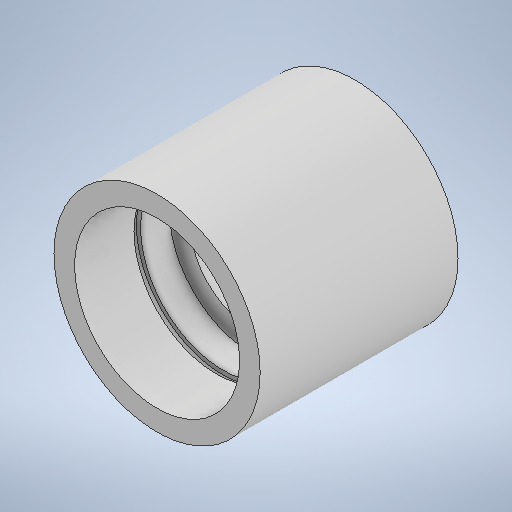
# Autodesk Inventor part: Седло для подшипника
Saved by Autodesk Inventor 2025 (Build 290162010, 162A)
## iProperties
Created: 2024-07-07
Part Number: Седло для подшипника
Material: Generic
Document SubType Name: Modeling
Designer: pokla
Density: 1 g/cm^3
Appearance: Default
Stock Number: Седло для подшипника
Author: pokla
Autodesk Inventor part; units mm, degrees
ref_plane "YZ Plane" through (0, 0, 0) normal (1, 0, 0) x (0, 1, 0)
ref_plane "XZ Plane" through (0, 0, 0) normal (0, 1, 0) x (-1, 0, 0)
ref_plane "XY Plane" through (0, 0, 0) normal (0, 0, 1) x (1, 0, 0)
sketch "Sketch6" plane through (0, 0, 0) normal (0, 0, 1) x (1, 0, 0)
  line L0 (20, 24) -> (25, 24)
  line L1 (25, 24) -> (25, -24)
  line L2 (25, -24) -> (20, -24)
  line L3 (20, -24) -> (20, -9.6)
  line L4 (15, 1) -> (20, 1)
  line L5 (20, 1) -> (20, -1) construction
  line L6 (20, -1) -> (15, -1)
  line L7 (15, -1) -> (15, 1)
  line L8 (20, -8) -> (21, -8)
  line L9 (21, -8) -> (21, -9.6)
  line L10 (21, -9.6) -> (20, -9.6)
  line L11 (20, -9.6) -> (20, -8) construction
  line L12 (20, 1) -> (20, 24)
  line L13 (20, -1) -> (20, 1) construction
  line L14 (20, -8) -> (20, -1)
  line L15 (20, -9.6) -> (20, -8) construction
  line L16 (0, -33.6) -> (0, 33.6) projected
  point P0 (0, 0)
  point P1 (25, 0)
  point P2 (20, 0)
  point P3 (20, -8.8)
  point P4 (20.5, -8)
  dimension "d12" = 48
  dimension "d13" = 25
  dimension "d14" = 5
  dimension "d15" = 2
  dimension "d16" = 5
  dimension "d17" = 7
  dimension "d18" = 1.6
  dimension "d19" = 1
  constraints: 32 end point, 10 parallel, 4 midpoint, 3 horizontal, 3 perpendicular, 2 horizontal alignment, 1 vertical alignment
  measures "d12" distance of L0.end L1.end
  measures "d13" distance from line of L1 point (0, 0)
  measures "d14" distance of L1.end L2.end
  measures "d15" distance of L6.end L4.start
  measures "d16" distance of L5.end L6.end
  measures "d17" distance from line of point (20.5, -8) L6
  measures "d18" distance of L8.end L9.end
  measures "d19" distance of L9.end L3.end
revolve "Revolution1" add sketch "Sketch6" angle 360 mid plane about axis through (0, -10, 0) along (0, 1, 0)
equation "\"d16\" = d14"
body "Solid2"
